# Autodesk Inventor part: JST-SH-03
Saved by Autodesk Inventor 2015 SP1 (Build 190203100, 203)
## iProperties
Created: 2015-10-19
Part Number: JST-SH-03
Material: Generic
Document SubType Name: Modeling
Designer: Kartikye
Density: 1 g/cm^3
Appearance: JST-SH-03, JST-SH-03
Author: Kartikye
Autodesk Inventor part; units mm, degrees
ref_plane "YZ Plane" through (0, 0, 0) normal (1, 0, 0) x (0, 1, 0)
ref_plane "XZ Plane" through (0, 0, 0) normal (0, 1, 0) x (-1, 0, 0)
ref_plane "XY Plane" through (0, 0, 0) normal (0, 0, 1) x (1, 0, 0)
sketch "JST-SH-03, JST-SH-03_100" plane through (0, 0, 0) normal (0, 0, 1) x (1, 0, 0)
  line L0 (-2.6635, 2.2) -> (2.6, 2.2)
  line L1 (2.6, 2.2) -> (2.6, -2.0635)
  line L2 (2.6, -2.0635) -> (-2.6635, -2.0635)
  line L3 (-2.6635, -2.0635) -> (-2.6635, 2.2)
  constraints: 8 end point
extrude "Extrusion1" add sketch "JST-SH-03, JST-SH-03_100" along normal blind 1
body "Solid1"
